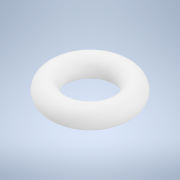
# Autodesk Inventor part: ToeSilikoneRubber
Saved by Autodesk Inventor 2022.2 (Build 262287000, 287)
## iProperties
Created: 2018-07-16
Part Number: ToeSilikoneRubber
Material: Generic
Document SubType Name: Modeling
Designer: Jochen
Density: 1 g/cm^3
Appearance: Default
Sending System: SolidWorks 2017
Last Author: Felix
Last Saved: 2021-02-23
Author: Jochen
Autodesk Inventor part; units mm, degrees
ref_plane "YZ Plane" through (0, 0, 0) normal (1, 0, 0) x (0, 1, 0)
ref_plane "XZ Plane" through (0, 0, 0) normal (0, 1, 0) x (-1, 0, 0)
ref_plane "XY Plane" through (0, 0, 0) normal (0, 0, 1) x (1, 0, 0)
sketch "Sketch1" plane through (0, 0, 0) normal (1, 0, 0) x (0, 1, 0)
  line L0 (0, -14.7) -> (0, 2.45) construction
  line L1 (-4.2, 0) -> (4.2, 0) construction
  circle A0 centre (0, -9.25) radius 3
  point P0 (0, 0)
  dimension "d0" = 6
  dimension "d2" = 9.25
  constraints: 1 centre point, 1 point on line
  measures "d0" diameter of A0
  measures "d2" distance of point (0, 0) A0.centre
revolve "Revolution1" add sketch "Sketch1" angle 360 about axis through (0, -10, 0) along (0, 1, 0)
body "Solid1"
body "Solid7"
